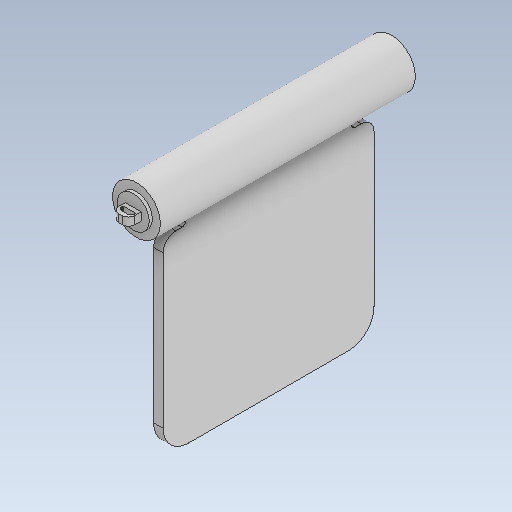
# Autodesk Inventor part: Ruder
Saved by Autodesk Inventor 2021 (Build 250183000, 183)
## iProperties
Created: 2021-01-08
Part Number: Ruder
Material: Generisch
Document SubType Name: Modeling
Designer: casa2
Density: 1 g/cm^3
Appearance: Vorgabe
Author: casa2
Autodesk Inventor part; units mm, degrees
ref_plane "YZ Plane" through (0, 0, 0) normal (1, 0, 0) x (0, 1, 0)
ref_plane "XZ Plane" through (0, 0, 0) normal (0, 1, 0) x (-1, 0, 0)
ref_plane "XY Plane" through (0, 0, 0) normal (0, 0, 1) x (1, 0, 0)
sketch "Skizze4" plane through (0, 0, 0) normal (0, 0, 1) x (1, 0, 0)
  circle A0 centre (0, 0) radius 7.5
  circle A1 centre (0, 0) radius 5
  dimension "d5" = 15
  dimension "d8" = 10
  constraints: 2 centre point, 2 coincident
  measures "d5" diameter of A0
  measures "d8" diameter of A1
extrude "Extrusion1" add sketch "Skizze4" along normal blind 80
sketch "Skizze5" plane through (0, 0, 0) normal (0, 1, 0) x (-1, 0, 0)
  line L0 (7.5, 80) -> (-7.5, 80) projected
  line L1 (7.5, 0) -> (-7.5, 0) projected
  line L2 (0, 0) -> (-3.4759, 0)
  line L3 (7.5, 0) -> (-7.5, 0) projected
  line L4 (0, 0) -> (0, 7)
  line L5 (7.5, 80) -> (-7.5, 80) projected
  line L6 (0, 80) -> (0, 73)
  line L7 (-5, 80) -> (-5, 0) projected
  line L8 (-1.5, 73.1365) -> (-1.5, 10.0002)
  line L9 (-7.5, 0) -> (-7.5, 80) projected
  line L10 (-1.5, 6.9605) -> (1.5, 6.9605)
  line L11 (5, 80) -> (5, 0) projected
  line L12 (1.5, 6.9605) -> (1.5, 73.1365)
  line L13 (1.5, 73.1365) -> (-1.566, 73.1365)
  line L14 (-1.5, 10.0002) -> (-1.5, 6.9605)
  point P0 (0, 70)
  dimension "d9" = 7
  dimension "d10" = 7
  dimension "d11" = 3
  constraints: 16 end point, 3 perpendicular, 3 point on line, 3 vertical, 1 midpoint, 1 parallel, 1 vertical alignment
  measures "d9" distance of L2.start L4.end
  measures "d10" distance of L6.start L6.end
  measures "d11" distance between parallel lines of L8 L12
extrude "Extrusion2" add sketch "Skizze5" along normal blind 1 and the other way blind 70 contours L13 L12 L10 L14 L8
sketch "Skizze7" plane through (0, 0, 80) normal (0, 0, 1) x (1, 0, 0)
  circle A0 centre (0, 0) radius 7.5 projected
  circle A1 centre (0, 0) radius 5 projected
  arc A2 (-1.5, -4.7697) -> (1.5, -4.7697) centre (0, 0) ccw projected
  line L0 (-1.5, 1) -> (1.5, 1) projected
  line L1 (-1.5, 1) -> (-1.5, -4.7697) projected
  line L2 (-1.5, -4.7697) -> (-1.5, 1) projected
  line L3 (-1.5, -4.7697) -> (-1.5, 1)
  line L4 (1.5, 1) -> (-1.5, 1) projected
  line L5 (-1.5, 1) -> (1.5, 1)
  line L6 (1.5, 1) -> (1.5, -4.7697)
  arc A3 (-1.5, -4.7697) -> (1.5, -4.7697) centre (0, 0) ccw projected
  arc A4 (-1.5, -4.7697) -> (1.5, -4.7697) centre (0, -2.7697) ccw
  line L7 (1.5, -4.7697) -> (1.5, 1) projected
  point P0 (-1.5, -4.7697)
  point P1 (1.5, -4.7697)
  point P2 (1.5, -4.7697)
  constraints: 6 end point, 2 collinear, 2 point on circle, 1 centre point, 1 perpendicular
extrude "Extrusion4" cut sketch "Skizze7" against normal blind 80 contours A1 L6 L0 L1 | L1 L0 L6 A1
sketch "Skizze8" plane through (1.5, -70, 73.1365) normal (1, 0, 0) x (0, 0, -1)
  line L0 (66.176, 62.6515) -> (0, 62.6515) projected
  line L1 (66.176, 0) -> (66.176, 62.6515) projected
  line L2 (0, 0) -> (66.176, 0) projected
  line L3 (0, 62.6515) -> (0, 0) projected
  line L4 (66.176, 62.6515) -> (0, 62.6515) projected
  line L5 (0, 62.6515) -> (7, 62.6515)
  line L6 (66.176, 62.5) -> (66.176, 62.6515) projected
  line L7 (66.176, 62.6515) -> (59.176, 62.6515)
  line L8 (7, 62.6515) -> (7, 59.6515)
  line L9 (33.088, 62.6515) -> (33.088, 0)
  line L10 (0, 0) -> (66.176, 0) projected
  line L11 (7, 59.6515) -> (0, 59.6515)
  line L12 (0, 62.6515) -> (0, 0) projected
  line L13 (0, 59.6515) -> (0, 0)
  line L14 (0, 0) -> (33.088, 0)
  line L15 (66.176, 0) -> (66.176, 62.6515)
  line L16 (59.176, 62.6515) -> (59.176, 59.6515)
  line L17 (59.176, 59.6515) -> (66.176, 59.6515)
  line L18 (66.176, 0) -> (33.088, 0)
  line L19 (7, 62.6515) -> (59.176, 62.6515)
  line L20 (0, 59.6515) -> (0, 62.6515)
  line L21 (66.176, 59.6515) -> (66.176, 62.5)
  point P0 (73.1365, 70)
  dimension "d20" = 7
  dimension "d21" = 7
  dimension "d22" = 3
  constraints: 28 end point, 5 collinear, 3 point on line, 2 midpoint, 2 symmetric about line, 2 vertical, 1 perpendicular
  measures "d20" distance of L0.end L5.end
  measures "d21" distance of L0.start L7.end
  measures "d22" distance of L5.end L8.end
extrude "Extrusion5" cut sketch "Skizze8" against normal blind 5 contours L1 L17 L16 L0 | L8 L11 L3 L0
fillet "Rundung7" radius 1 4 edges at (0, -7.3485, 66.1365) (0, -10.3485, 66.1365) (0, -7.3485, 13.9605) (0, -10.3485, 13.9605)
fillet "Rundung8" radius 4 2 edges at (0, -10.3485, 6.9605) (0, -10.3485, 73.1365)
fillet "Rundung9" radius 8 2 edges at (0, -70, 73.1365) (0, -70, 6.9605)
sketch "Skizze9" plane through (0, 0, 80) normal (0, 0, 1) x (1, 0, 0)
  circle A0 centre (0, 0) radius 7.5 projected
  circle A1 centre (0, 0) radius 5 projected
  circle A2 centre (0, 0) radius 5
  line L0 (2.5, 1.25) -> (-2.5, 1.25)
  line L1 (-2.5, 1.25) -> (-2.5, -1.25)
  line L2 (-2.5, -1.25) -> (2.5, -1.25)
  line L3 (2.5, -1.25) -> (2.5, 1.25)
  line L4 (0, 1.25) -> (0, -1.25)
  dimension "d37" = 10
  dimension "d38" = 5
  dimension "d39" = 2.5
  constraints: 10 end point, 3 coincident, 3 midpoint, 2 parallel, 1 centre point, 1 horizontal, 1 perpendicular
  measures "d37" diameter of A2
  measures "d38" distance of L2.end L1.end
  measures "d39" distance of L1.end L0.end
extrude "Extrusion6" add sketch "Skizze9" along normal blind 1 contours A1
extrude "Extrusion7" add sketch "Skizze9" along normal blind 5 contours L3 L2 L4 L0 | L4 L2 L1 L0
sketch "Skizze10" plane through (-2.5, -1.25, 81) normal (0, -1, 0) x (1, 0, 0)
  line L0 (0, 0) -> (5, 0) projected
  line L1 (0, 0) -> (0, 4) projected
  line L2 (5, 4) -> (0, 4) projected
  line L3 (5, 0) -> (5, 4) projected
  line L4 (5, 4) -> (0, 4) projected
  line L5 (7.5, 0) -> (-2.5, 0) projected
  line L6 (0, 0) -> (0, 4) projected
  line L7 (5, 0) -> (5, 4) projected
  line L8 (0.5, 2.75) -> (4.5, 2.75)
  line L9 (4.5, 2.75) -> (4.5, 1.25)
  line L10 (4.5, 1.25) -> (0.5, 1.25)
  line L11 (0.5, 1.25) -> (0.5, 2.75)
  line L12 (2.5, 4) -> (2.5, 0)
  line L13 (0.5, 2) -> (4.5, 2)
  point P0 (2.5, -81)
  point P1 (2.5, 2)
  point P2 (2.5, 2)
  dimension "d44" = 4
  dimension "d45" = 1.5
  constraints: 12 end point, 6 midpoint, 2 coincident, 2 parallel, 1 horizontal, 1 perpendicular
  measures "d44" distance of L9.end L10.end
  measures "d45" distance of L8.end L9.end
extrude "Extrusion8" cut sketch "Skizze10" against normal blind 5 contours L12 L13 L9 L10 | L10 L11 L13 L12 | L13 L11 L8 L12 | L12 L8 L9 L13
fillet "Rundung10" radius 2 2 edges at (-2.5, 0, 85) (2.5, 0, 85)
fillet "Rundung11" radius 1 1 edges at (-2, 0, 83.75)
fillet "Rundung11" radius 1 1 edges at (2, 0, 83.75)
fillet "Rundung12" radius 0.2 1 edges at (2, 0, 82.25)
fillet "Rundung12" radius 0.2 1 edges at (-2, 0, 82.25)
equation "\"d5\" = Durchmesser1"
equation "\"d8\" = Durchmesser3"
equation "\"d6\" = Länge1"
equation "\"d9\" = Größe1"
equation "\"d10\" = Größe1"
equation "\"d11\" = Durchmesser2"
equation "\"d13\" = Größe2"
equation "\"d20\" = Größe1"
equation "\"d21\" = Größe1"
equation "\"d22\" = Größe3"
equation "\"Durchmesser1\" = 15"
equation "\"Länge1\" = 80"
equation "\"Größe1\" = 7"
equation "\"Durchmesser2\" = 3"
equation "\"Durchmesser3\" = 10"
equation "\"Größe2\" = 70"
equation "\"Größe3\" = 3"
equation "\"Größe4\" = 15"
